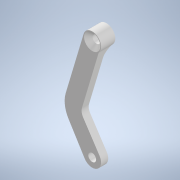
# Autodesk Inventor part: lidar_shatun_main2
Saved by Autodesk Inventor 2022 (Build 260153000, 153)
## iProperties
Created: 2024-10-21
Part Number: lidar_shatun_main2
Material: Типовые
Document SubType Name: Modeling
Designer: Andrey
Density: 1 g/cm^3
Appearance: По умолчанию
Author: Andrey
Autodesk Inventor part; units mm, degrees
ref_plane "YZ Plane" through (0, 0, 0) normal (1, 0, 0) x (0, 1, 0)
ref_plane "XZ Plane" through (0, 0, 0) normal (0, 1, 0) x (-1, 0, 0)
ref_plane "XY Plane" through (0, 0, 0) normal (0, 0, 1) x (1, 0, 0)
sketch "Эскиз1" plane through (0, 0, 0) normal (0, 0, 1) x (1, 0, 0)
  line L0 (3.25, -11.7591) -> (3.25, 11.7591)
  arc A0 (3.25, 11.7591) -> (-0.577, 12.5728) centre (1.25, 11.7591) ccw
  arc A1 (-0.577, 12.5728) -> (-0.577, -12.5728) centre (27.6554, 0) ccw
  arc A2 (-0.577, -12.5728) -> (3.25, -11.7591) centre (1.25, -11.7591) ccw
  circle A3 centre (0, 0) radius 1.6
  arc A4 (6.4668, 10.3451) -> (3.0304, 12.2157) centre (4.5497, 10.9151) ccw
  line L1 (8.1572, 16.0299) -> (6.4668, 10.3451)
  spline S0 degree 3 poles (10.4238, 16.9209) (10.1757, 16.9946) (9.8678, 17.0343) (9.3849, 17.0076) (9.1215, 16.949) (8.7408, 16.7764) (8.5508, 16.6436) (8.3079, 16.3721) (8.206, 16.1939) (8.1572, 16.0299) knots 0 0 0 0 0.305206 0.305206 0.570377 0.570377 0.79822 0.79822 1 1 1 1
  line L2 (10.4238, 16.9209) -> (14.341, 15.7561)
  line L3 (14.9111, 17.6731) -> (14.341, 15.7561)
  line L4 (14.9111, 17.6731) -> (2.8821, 21.25)
  arc A5 (2.8821, 21.25) -> (-9.197, -19.3722) centre (26.5083, -7.8823) ccw
  line L5 (2.8319, -22.949) -> (-9.197, -19.3722)
  line L6 (3.402, -21.032) -> (2.8319, -22.949)
  line L7 (3.402, -21.032) -> (-0.5153, -19.8672)
  spline S1 degree 3 poles (-1.9268, -17.8826) (-1.9756, -18.0465) (-1.9876, -18.2515) (-1.9324, -18.6116) (-1.8459, -18.8266) (-1.6213, -19.1792) (-1.4327, -19.3722) (-1.0429, -19.6584) (-0.7633, -19.7934) (-0.5153, -19.8672) knots 0 0 0 0 0.20178 0.20178 0.429623 0.429623 0.694794 0.694794 1 1 1 1
  line L8 (-0.2364, -12.1977) -> (-1.9268, -17.8826)
  arc A6 (-4.1366, -11.8868) -> (-0.2364, -12.1977) centre (-2.1534, -11.6276) ccw
  arc A7 (3.0304, 12.2157) -> (-4.1366, -11.8868) centre (26.5083, -7.8823) ccw
  arc A8 (-3.8043, 5.6518) -> (-6.5436, 6.8749) centre (-5.174, 6.2633) ccw
  arc A9 (-3.8043, 5.6518) -> (-6.2743, -2.6549) centre (26.5083, -7.8823) ccw
  arc A10 (-9.2369, -2.1825) -> (-6.2743, -2.6549) centre (-7.7556, -2.4187) ccw
  arc A11 (-6.5436, 6.8749) -> (-9.2369, -2.1825) centre (26.5083, -7.8823) ccw
  line L9 (-0.2364, -12.1977) -> (6.4668, 10.3451)
  arc A12 (6.4668, 10.3451) -> (3.0304, 12.2157) centre (4.5497, 10.9151) ccw
  arc A13 (3.0304, 12.2157) -> (-4.1366, -11.8868) centre (26.5083, -7.8823) ccw
  arc A14 (-4.1366, -11.8868) -> (-0.2364, -12.1977) centre (-2.1534, -11.6276) ccw
  circle A15 centre (0, 0) radius 1.6
  arc A16 (-12.224, -21.5992) -> (-13.8334, -29.3505) centre (-13.5929, -25.3577) ccw
  line L10 (-13.8334, -29.3505) -> (-0.1202, -30.1764)
  arc A17 (-0.1202, -30.1764) -> (0.6845, -26.3008) centre (0, -28.18) ccw
  line L11 (0.6845, -26.3008) -> (-12.224, -21.5992)
  circle A18 centre (0, -28.18) radius 1.1
  circle A19 centre (-13.5929, -25.3577) radius 1.9
  line L12 (0, 0) -> (0, -28.18)
  circle A20 centre (0, -28.18) radius 1.1
  circle A21 centre (0, 0) radius 1.1
  circle A22 centre (0, 0) radius 2.5
  circle A23 centre (0, -28.18) radius 2.5
  arc A24 (6.4668, 10.3451) -> (3.0304, 12.2157) centre (4.5497, 10.9151) ccw
  line L13 (8.1572, 16.0299) -> (6.4668, 10.3451)
  spline S2 degree 3 poles (10.4238, 16.9209) (10.1757, 16.9946) (9.8678, 17.0343) (9.3849, 17.0076) (9.1215, 16.949) (8.7408, 16.7764) (8.5508, 16.6436) (8.3079, 16.3721) (8.206, 16.1939) (8.1572, 16.0299) knots 0 0 0 0 0.305206 0.305206 0.570377 0.570377 0.79822 0.79822 1 1 1 1
  line L14 (10.4238, 16.9209) -> (14.341, 15.7561)
  line L15 (14.9111, 17.6731) -> (14.341, 15.7561)
  line L16 (14.9111, 17.6731) -> (2.8821, 21.25)
  arc A25 (2.8821, 21.25) -> (-9.197, -19.3722) centre (26.5083, -7.8823) ccw
  line L17 (2.8319, -22.949) -> (-9.197, -19.3722)
  line L18 (3.402, -21.032) -> (2.8319, -22.949)
  line L19 (3.402, -21.032) -> (-0.5153, -19.8672)
  spline S3 degree 3 poles (-1.9268, -17.8826) (-1.9756, -18.0465) (-1.9876, -18.2515) (-1.9324, -18.6116) (-1.8459, -18.8266) (-1.6213, -19.1792) (-1.4327, -19.3722) (-1.0429, -19.6584) (-0.7633, -19.7934) (-0.5153, -19.8672) knots 0 0 0 0 0.20178 0.20178 0.429623 0.429623 0.694794 0.694794 1 1 1 1
  line L20 (-0.2364, -12.1977) -> (-1.9268, -17.8826)
  arc A26 (-4.1366, -11.8868) -> (-0.2364, -12.1977) centre (-2.1534, -11.6276) ccw
  arc A27 (3.0304, 12.2157) -> (-4.1366, -11.8868) centre (26.5083, -7.8823) ccw
  arc A28 (-3.8043, 5.6518) -> (-6.5436, 6.8749) centre (-5.174, 6.2633) ccw
  arc A29 (-3.8043, 5.6518) -> (-6.2743, -2.6549) centre (26.5083, -7.8823) ccw
  arc A30 (-9.2369, -2.1825) -> (-6.2743, -2.6549) centre (-7.7556, -2.4187) ccw
  arc A31 (-6.5436, 6.8749) -> (-9.2369, -2.1825) centre (26.5083, -7.8823) ccw
  line L21 (-1.1949, -11.9127) -> (-2.8853, -17.5975)
  line L22 (2.0911, -26.8099) -> (-2.5802, -19.6802)
  line L23 (-2.8853, -17.5975) -> (1.8461, -1.6858)
  circle A32 centre (-0.489, -18.3101) radius 2.5
  circle A33 centre (-0.489, -18.3101) radius 1.5
  line L24 (-7.4383, -16.2437) -> (-2.3963, 0.7125)
  circle A34 centre (-0.489, -18.3101) radius 7.25
  line L25 (-2.1301, -29.4887) -> (-6.6663, -22.1053)
  dimension "d14" = 28.18
  dimension "d15" = 2.2
  dimension "d16" = 2.2
  dimension "d17" = 5
  dimension "d18" = 5
  dimension "d19" = 1
  constraints: 12 end point, 8 point on circle, 7 tangent, 6 centre point, 6 coincident, 2 parallel, 1 collinear, 1 vertical, 5 other
  measures "d14" distance of L12.start L12.end
  measures "d15" diameter of A20
  measures "d16" diameter of A21
  measures "d17" diameter of A22
  measures "d18" diameter of A23
  measures "d19" distance between parallel lines of L8 L21
extrude "Выдавливание1" add sketch "Эскиз1" along normal blind 2 contours A34 L12 L22 | L22 A23 L12 A34 | L23 A34 A1 L24 A22 L12 | L12 A22 L23 | L23 A1 A34 | A23 L10 A17 L11 L12 | L12 A34 L11 L5 L22 | L12 A23 L11 A34 | A22 | L23 L21 A6 A34 A1 | A34 A6 A7 L24 A1 | L21 A32 L22 L5 A34 A6 | L12 L11 A23 | A34 L11 | L11 A23 L25 A34 | A7 A6 A34 L24 | A23 L11 A17 L10 | L11 L25 A34 | A3
sketch "Эскиз2" plane through (0, 0, 0) normal (0, 0, -1) x (-1, 0, 0)
  line L0 (2.3963, 0.7125) -> (7.4383, -16.2437) projected
  arc A0 (2.3963, 0.7125) -> (-1.8461, -1.6858) centre (0, 0) ccw projected
  line L1 (2.8853, -17.5975) -> (-1.8461, -1.6858) projected
  arc A1 (2.5802, -19.6802) -> (2.8853, -17.5975) centre (0.489, -18.3101) ccw projected
  line L2 (-2.0911, -26.8099) -> (2.5802, -19.6802) projected
  arc A2 (-2.0911, -26.8099) -> (2.1301, -29.4887) centre (0, -28.18) ccw projected
  line L3 (6.6663, -22.1053) -> (2.1301, -29.4887) projected
  arc A3 (6.6663, -22.1053) -> (7.4383, -16.2437) centre (0.489, -18.3101) ccw projected
  circle A4 centre (0, 0) radius 1.1 projected
  circle A5 centre (0, -28.18) radius 1.1 projected
  circle A6 centre (0, 0) radius 2.5
  point P0 (0, 0)
  constraints: 1 coincident, 3 other
extrude "Выдавливание2" add sketch "Эскиз2" along normal blind 2 contours A6 A0
fillet "Сопряжение3" radius 2 1 edges at (-1.2303, -2.1763, 0)
fillet "Сопряжение4" radius 2 2 edges at (1.8461, -1.6858, 1) (1.8461, -1.6858, -1)
chamfer "Фаска1" distance 1.2 angle 45 1 edges at (-1.1, 0, 2)
